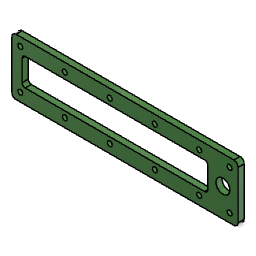
3d06 v1 (Autodesk Fusion 360 design; units mm, degrees)
Autodesk Fusion 360 part; units mm, degrees
sketch "Sketch1" plane through (0, 0, 0) normal (0, 0, 1) x (1, 0, 0)
  line L0 (0.5, 0) -> (30, 0)
  line L1 (30.5, 0.5) -> (30.5, 4)
  line L2 (30, 4.5) -> (0.5, 4.5)
  line L3 (0, 4) -> (0, 0.5)
  arc A0 (0, 0.5) -> (0.5, 0) centre (0.5, 0.5) ccw
  arc A1 (0.5, 4.5) -> (0, 4) centre (0.5, 4) ccw
  arc A2 (30.5, 4) -> (30, 4.5) centre (30, 4) ccw
  arc A3 (30, 0) -> (30.5, 0.5) centre (30, 0.5) ccw
  line L4 (-18.1072, 2.25) -> (79.1072, 2.25) construction
  circle A4 centre (14.4, -1) radius 0.4
  circle A5 centre (-0.3, -1) radius 0.4
  circle A6 centre (7, -1) radius 0.4
  circle A7 centre (21.8, -1) radius 0.4
  circle A8 centre (29.1, -1) radius 0.4
  circle A9 centre (34.1, -1) radius 0.4
  line L5 (-2.117, -1) -> (37.883, -1) construction
  circle A10 centre (34.1, 5.5) radius 0.4
  circle A11 centre (29.1, 5.5) radius 0.4
  circle A12 centre (21.8, 5.5) radius 0.4
  circle A13 centre (14.4, 5.5) radius 0.4
  circle A14 centre (7, 5.5) radius 0.4
  circle A15 centre (-0.3, 5.5) radius 0.4
  line L6 (24, 2.25) -> (37, 2.25) construction
  line L7 (33, 4.7661) -> (33, -0.2339)
  line L8 (-1, 6.9) -> (34.8, 6.9)
  line L9 (35.5, 6.2) -> (35.5, -1.7)
  line L10 (34.8, -2.4) -> (-1, -2.4)
  line L11 (-1.7, -1.7) -> (-1.7, 6.2)
  arc A16 (-1, 6.9) -> (-1.7, 6.2) centre (-1, 6.2) ccw
  arc A17 (-1.7, -1.7) -> (-1, -2.4) centre (-1, -1.7) ccw
  arc A18 (34.8, -2.4) -> (35.5, -1.7) centre (34.8, -1.7) ccw
  arc A19 (35.5, 6.2) -> (34.8, 6.9) centre (34.8, 6.2) ccw
  circle A20 centre (33, 2.2661) radius 1.15
  point P0 (30.5, 0)
  point P1 (0, 4.5)
  point P2 (-1.7, 6.9)
  point P3 (35.5, 6.9)
  point P4 (-1.7, -2.4)
  dimension "d1" = 30.5
  dimension "d2" = 4.5
  dimension "d3" = 0.5
  dimension "d4" = 0.5
  dimension "d5" = 0.5
  dimension "d6" = 0.5
  dimension "d7" = 0.8
  dimension "d8" = 0.8
  dimension "d9" = 0.8
  dimension "d10" = 0.8
  dimension "d11" = 0.8
  dimension "d12" = 0.8
  dimension "d13" = 5
  dimension "d14" = 12.3
  dimension "d15" = 19.7
  dimension "d16" = 27.1
  dimension "d17" = 34.4
  dimension "d18" = 3.6
  dimension "d20" = 5.5
  dimension "d21" = 6.5
  dimension "d22" = 37.2
  dimension "d23" = 9.3
  dimension "d24" = 1.4
  dimension "d25" = 1.4
  dimension "d27" = 1.4
  dimension "d28" = 0.7
  dimension "d29" = 0.7
  dimension "d30" = 0.7
  dimension "d31" = 0.7
  dimension "d32" = 2.5
  dimension "d33" = 2.3
  dimension "d34" = 33.4598
  constraint horizontal L0
  constraint vertical L1
  constraint horizontal L2
  constraint vertical L3
  constraint coincident origin L0
  constraint coincident origin L3
  constraint tangent L0 A0
  constraint tangent L3 A0
  constraint coincident P1 L2
  constraint coincident P1 L3
  constraint tangent L2 A1
  constraint tangent L3 A1
  constraint tangent L1 A2
  constraint tangent L2 A2
  constraint coincident P0 L0
  constraint coincident P0 L1
  constraint tangent L0 A3
  constraint tangent L1 A3
  constraint horizontal L4
  constraint midpoint L1 L4
  constraint horizontal L5
  constraint coincident A5.centre L5
  constraint coincident A4.centre L5
  constraint coincident A7.centre L5
  constraint coincident A8.centre L5
  constraint coincident A9.centre L5
  constraint coincident A6.centre L5
  constraint symmetric L4 A4 A13
  constraint symmetric L4 A5 A15
  constraint symmetric L4 A6 A14
  constraint symmetric L4 A7 A12
  constraint symmetric L4 A8 A11
  constraint symmetric L4 A9 A10
  constraint horizontal L6
  constraint perpendicular L6 L7
  constraint midpoint L1 L6
  constraint horizontal L8
  constraint vertical L9
  constraint horizontal L10
  constraint vertical L11
  constraint coincident P4 L10
  constraint coincident P2 L11
  constraint tangent L8 A16
  constraint tangent L11 A16
  constraint coincident P4 L11
  constraint tangent L11 A17
  constraint tangent L10 A17
  constraint tangent L10 A18
  constraint tangent L9 A18
  constraint coincident P3 L8
  constraint coincident P3 L9
  constraint tangent L8 A19
  constraint tangent L9 A19
  constraint midpoint L7 A20.centre
  measures "d1" distance of origin P0
  measures "d2" distance of origin P1
  measures "d3" radius of A0
  measures "d4" radius of A1
  measures "d5" radius of A2
  measures "d6" radius of A3
  measures "d7" diameter of A4
  measures "d8" diameter of A5
  measures "d9" diameter of A6
  measures "d10" diameter of A7
  measures "d11" diameter of A8
  measures "d12" diameter of A9
  measures "d13" distance of A8.centre A9.centre
  measures "d14" distance of A7.centre A9.centre
  measures "d15" distance of A4.centre A9.centre
  measures "d16" distance of A6.centre A9.centre
  measures "d17" distance of A5.centre A9.centre
  measures "d18" distance of L1 A9.centre
  measures "d20" vertical distance of P0 A10.centre
  measures "d21" distance of A9.centre A10.centre
  measures "d22" distance of P2 P3
  measures "d23" distance of P2 P4
  measures "d24" distance of A10.centre L9
  measures "d25" distance of A10.centre L8
  measures "d27" distance of A9.centre L10
  measures "d28" radius of A16
  measures "d29" radius of A17
  measures "d30" radius of A18
  measures "d31" radius of A19
  measures "d32" distance of L7 L9
  measures "d33" diameter of A20
  measures "d34" distance of A5.centre A20.centre
extrude "Extrude1" add sketch "Sketch1" along normal mid plane 1
